Autodesk Inventor part; units mm, degrees
(part 6 of 6)
sketch "スケッチ6" plane through (0, 0, 3) normal (0, 0, 1) x (1, 0, 0)
  arc A0 (23.1244, 53.4347) -> (21.933, 55.8475) centre (21.2019, 53.9859) ccw projected
  arc A1 (21.933, 55.8475) -> (10.9945, 58.9841) centre (0, 0) ccw projected
  arc A2 (10.9945, 58.9841) -> (8.7055, 57.5692) centre (10.628, 57.0179) ccw projected
  line L0 (8.7055, 57.5692) -> (4.5912, 43.221) projected
  arc A3 (3.3812, 41.9035) -> (4.5912, 43.221) centre (2.6687, 43.7723) ccw projected
  line L1 (3.3812, 41.9035) -> (-9.7193, 36.9085) projected
  arc A4 (-12.3349, 38.1621) -> (-9.7193, 36.9085) centre (-10.4318, 38.7772) ccw projected
  line L2 (-12.3349, 38.1621) -> (-15.32, 47.3978) projected
  line L3 (-15.32, 47.3978) -> (-15.6651, 47.2849) projected
  line L4 (-15.6651, 47.2849) -> (-16.0093, 47.1694) projected
  line L5 (-16.0093, 47.1694) -> (-16.3527, 47.0515) projected
  line L6 (-16.3527, 47.0515) -> (-16.6952, 46.9311) projected
  line L7 (-16.6952, 46.9311) -> (-17.0368, 46.8081) projected
  line L8 (-17.0368, 46.8081) -> (-17.3775, 46.6827) projected
  line L9 (-17.3775, 46.6827) -> (-17.7172, 46.5548) projected
  line L10 (-17.7172, 46.5548) -> (-18.0561, 46.4245) projected
  line L11 (-18.0561, 46.4245) -> (-18.394, 46.2916) projected
  line L12 (-18.394, 46.2916) -> (-18.7309, 46.1563) projected
  line L13 (-18.7309, 46.1563) -> (-18.8024, 45.721) projected
  line L14 (-18.8024, 45.721) -> (-18.866, 45.2878) projected
  line L15 (-18.866, 45.2878) -> (-18.9216, 44.8569) projected
  line L16 (-18.9216, 44.8569) -> (-18.969, 44.4283) projected
  line L17 (-18.969, 44.4283) -> (-19.0083, 44.0023) projected
  line L18 (-19.0083, 44.0023) -> (-19.0392, 43.579) projected
  line L19 (-19.0392, 43.579) -> (-19.0617, 43.1585) projected
  line L20 (-19.0617, 43.1585) -> (-19.0757, 42.7409) projected
  line L21 (-19.0757, 42.7409) -> (-19.081, 42.3265) projected
  line L22 (-19.081, 42.3265) -> (-19.0774, 41.9154) projected
  line L23 (-19.0774, 41.9154) -> (-19.0647, 41.5079) projected
  line L24 (-19.0647, 41.5079) -> (-19.0425, 41.1041) projected
  line L25 (-19.0425, 41.1041) -> (-19.0107, 40.7043) projected
  line L26 (-19.0107, 40.7043) -> (-18.9686, 40.3088) projected
  line L27 (-18.9686, 40.3088) -> (-18.9158, 39.9179) projected
  line L28 (-18.9158, 39.9179) -> (-18.8516, 39.5322) projected
  line L29 (-18.8516, 39.5322) -> (-18.7748, 39.1522) projected
  line L30 (-18.7748, 39.1522) -> (-18.6839, 38.7788) projected
  line L31 (-18.6839, 38.7788) -> (-18.576, 38.4134) projected
  line L32 (-18.576, 38.4134) -> (-18.4431, 38.0601) projected
  line L33 (-18.4431, 38.0601) -> (-18.3313, 37.804) projected
  line L34 (-18.3313, 37.804) -> (-18.2337, 37.5507) projected
  line L35 (-18.2337, 37.5507) -> (-18.1486, 37.3012) projected
  line L36 (-18.1486, 37.3012) -> (-18.0734, 37.0569) projected
  line L37 (-18.0734, 37.0569) -> (-18.0133, 36.8155) projected
  line L38 (-18.0133, 36.8155) -> (-17.9685, 36.5772) projected
  line L39 (-17.9685, 36.5772) -> (-17.9393, 36.342) projected
  line L40 (-17.9393, 36.342) -> (-17.9202, 36.1129) projected
  line L41 (-17.9202, 36.1129) -> (-17.9169, 35.8874) projected
  line L42 (-17.9169, 35.8874) -> (-17.9314, 35.6648) projected
  line L43 (-17.9314, 35.6648) -> (-17.9574, 35.4486) projected
  line L44 (-17.9574, 35.4486) -> (-18.0008, 35.2362) projected
  line L45 (-18.0008, 35.2362) -> (-18.0614, 35.0282) projected
  line L46 (-18.0614, 35.0282) -> (-18.1365, 34.8267) projected
  line L47 (-18.1365, 34.8267) -> (-18.2329, 34.6288) projected
  line L48 (-18.2329, 34.6288) -> (-18.3447, 34.4386) projected
  line L49 (-18.3447, 34.4386) -> (-18.4826, 34.2517) projected
  line L50 (-18.4826, 34.2517) -> (-18.6427, 34.0722) projected
  line L51 (-18.6427, 34.0722) -> (-18.8473, 33.8913) projected
  line L52 (-18.8473, 33.8913) -> (-19.1345, 33.6962) projected
  line L53 (-19.1345, 33.6962) -> (-19.1827, 33.6688) projected
  line L54 (-19.1827, 33.6688) -> (-19.2308, 33.6413) projected
  line L55 (-19.2308, 33.6413) -> (-19.2789, 33.6138) projected
  line L56 (-19.2789, 33.6138) -> (-19.327, 33.5862) projected
  line L57 (-19.327, 33.5862) -> (-19.375, 33.5585) projected
  line L58 (-19.375, 33.5585) -> (-19.423, 33.5307) projected
  line L59 (-19.423, 33.5307) -> (-19.4709, 33.5029) projected
  line L60 (-19.4709, 33.5029) -> (-19.5188, 33.475) projected
  line L61 (-19.5188, 33.475) -> (-19.5667, 33.4471) projected
  line L62 (-19.5667, 33.4471) -> (-19.6145, 33.4191) projected
  line L63 (-19.6145, 33.4191) -> (-19.9271, 33.2679) projected
  line L64 (-19.9271, 33.2679) -> (-20.186, 33.1812) projected
  line L65 (-20.186, 33.1812) -> (-20.4215, 33.1323) projected
  line L66 (-20.4215, 33.1323) -> (-20.6524, 33.1063) projected
  line L67 (-20.6524, 33.1063) -> (-20.8729, 33.1046) projected
  line L68 (-20.8729, 33.1046) -> (-21.0926, 33.12) projected
  line L69 (-21.0926, 33.12) -> (-21.3046, 33.1558) projected
  line L70 (-21.3046, 33.1558) -> (-21.515, 33.2073) projected
  line L71 (-21.515, 33.2073) -> (-21.7207, 33.2758) projected
  line L72 (-21.7207, 33.2758) -> (-21.9209, 33.3615) projected
  line L73 (-21.9209, 33.3615) -> (-22.121, 33.4602) projected
  line L74 (-22.121, 33.4602) -> (-22.3146, 33.5758) projected
  line L75 (-22.3146, 33.5758) -> (-22.5034, 33.7069) projected
  line L76 (-22.5034, 33.7069) -> (-22.6925, 33.8498) projected
  line L77 (-22.6925, 33.8498) -> (-22.8765, 34.0078) projected
  line L78 (-22.8765, 34.0078) -> (-23.0555, 34.1805) projected
  line L79 (-23.0555, 34.1805) -> (-23.2294, 34.3678) projected
  line L80 (-23.2294, 34.3678) -> (-23.403, 34.5662) projected
  line L81 (-23.403, 34.5662) -> (-23.5736, 34.7774) projected
  line L82 (-23.5736, 34.7774) -> (-23.7394, 35.0022) projected
  line L83 (-23.7394, 35.0022) -> (-23.979, 35.294) projected
  line L84 (-23.979, 35.294) -> (-24.2415, 35.5701) projected
  line L85 (-24.2415, 35.5701) -> (-24.5194, 35.8356) projected
  line L86 (-24.5194, 35.8356) -> (-24.8101, 36.092) projected
  line L87 (-24.8101, 36.092) -> (-25.1121, 36.3405) projected
  line L88 (-25.1121, 36.3405) -> (-25.4241, 36.5817) projected
  line L89 (-25.4241, 36.5817) -> (-25.7456, 36.8158) projected
  line L90 (-25.7456, 36.8158) -> (-26.0759, 37.0434) projected
  line L91 (-26.0759, 37.0434) -> (-26.4145, 37.2644) projected
  line L92 (-26.4145, 37.2644) -> (-26.7611, 37.4792) projected
  line L93 (-26.7611, 37.4792) -> (-27.1153, 37.6879) projected
  line L94 (-27.1153, 37.6879) -> (-27.4768, 37.8905) projected
  line L95 (-27.4768, 37.8905) -> (-27.8455, 38.0872) projected
  line L96 (-27.8455, 38.0872) -> (-28.2209, 38.2779) projected
  line L97 (-28.2209, 38.2779) -> (-28.603, 38.4628) projected
  line L98 (-28.603, 38.4628) -> (-28.9916, 38.6418) projected
  line L99 (-28.9916, 38.6418) -> (-29.3864, 38.815) projected
  line L100 (-29.3864, 38.815) -> (-29.7874, 38.9823) projected
  line L101 (-29.7874, 38.9823) -> (-30.1943, 39.1439) projected
  line L102 (-30.1943, 39.1439) -> (-30.6071, 39.2996) projected
  line L103 (-30.6071, 39.2996) -> (-30.8927, 39.0755) projected
  line L104 (-30.8927, 39.0755) -> (-31.1767, 38.8493) projected
  line L105 (-31.1767, 38.8493) -> (-31.459, 38.621) projected
  line L106 (-31.459, 38.621) -> (-31.7397, 38.3907) projected
  line L107 (-31.7397, 38.3907) -> (-32.0186, 38.1583) projected
  line L108 (-32.0186, 38.1583) -> (-32.2959, 37.924) projected
  line L109 (-32.2959, 37.924) -> (-32.5715, 37.6876) projected
  line L110 (-32.5715, 37.6876) -> (-32.8453, 37.4492) projected
  line L111 (-32.8453, 37.4492) -> (-33.1173, 37.2088) projected
  line L112 (-33.1173, 37.2088) -> (-33.3877, 36.9664) projected
  line L113 (-33.3877, 36.9664) -> (-33.306, 36.5329) projected
  line L114 (-33.306, 36.5329) -> (-33.2176, 36.1041) projected
  line L115 (-33.2176, 36.1041) -> (-33.1224, 35.6801) projected
  line L116 (-33.1224, 35.6801) -> (-33.0204, 35.2612) projected
  line L117 (-33.0204, 35.2612) -> (-32.9116, 34.8475) projected
  line L118 (-32.9116, 34.8475) -> (-32.7959, 34.4391) projected
  line L119 (-32.7959, 34.4391) -> (-32.6732, 34.0362) projected
  line L120 (-32.6732, 34.0362) -> (-32.5436, 33.639) projected
  line L121 (-32.5436, 33.639) -> (-32.4068, 33.2478) projected
  line L122 (-32.4068, 33.2478) -> (-32.2628, 32.8628) projected
  line L123 (-32.2628, 32.8628) -> (-32.1115, 32.4841) projected
  line L124 (-32.1115, 32.4841) -> (-31.9525, 32.1123) projected
  line L125 (-31.9525, 32.1123) -> (-31.7858, 31.7475) projected
  line L126 (-31.7858, 31.7475) -> (-31.6111, 31.3902) projected
  line L127 (-31.6111, 31.3902) -> (-31.4278, 31.041) projected
  line L128 (-31.4278, 31.041) -> (-31.2355, 30.7005) projected
  line L129 (-31.2355, 30.7005) -> (-31.0334, 30.3697) projected
  line L130 (-31.0334, 30.3697) -> (-30.8202, 30.0499) projected
  line L131 (-30.8202, 30.0499) -> (-30.5939, 29.7434) projected
  line L132 (-30.5939, 29.7434) -> (-30.3482, 29.4569) projected
  line L133 (-30.3482, 29.4569) -> (-30.1555, 29.2545) projected
  line L134 (-30.1555, 29.2545) -> (-29.9772, 29.0498) projected
  line L135 (-29.9772, 29.0498) -> (-29.8119, 28.8444) projected
  line L136 (-29.8119, 28.8444) -> (-29.6577, 28.6406) projected
  line L137 (-29.6577, 28.6406) -> (-29.5186, 28.4343) projected
  line L138 (-29.5186, 28.4343) -> (-29.395, 28.2257) projected
  line L139 (-29.395, 28.2257) -> (-29.2872, 28.0147) projected
  line L140 (-29.2872, 28.0147) -> (-29.1908, 27.806) projected
  line L141 (-29.1908, 27.806) -> (-29.1106, 27.5952) projected
  line L142 (-29.1106, 27.5952) -> (-29.0481, 27.381) projected
  line L143 (-29.0481, 27.381) -> (-28.9985, 27.169) projected
  line L144 (-28.9985, 27.169) -> (-28.9667, 26.9545) projected
  line L145 (-28.9667, 26.9545) -> (-28.9525, 26.7384) projected
  line L146 (-28.9525, 26.7384) -> (-28.9541, 26.5234) projected
  line L147 (-28.9541, 26.5234) -> (-28.9771, 26.3044) projected
  line L148 (-28.9771, 26.3044) -> (-29.0171, 26.0875) projected
  line L149 (-29.0171, 26.0875) -> (-29.0828, 25.8646) projected
  line L150 (-29.0828, 25.8646) -> (-29.1718, 25.6412) projected
  line L151 (-29.1718, 25.6412) -> (-29.3021, 25.4012) projected
  line L152 (-29.3021, 25.4012) -> (-29.5054, 25.1196) projected
  line L153 (-29.5054, 25.1196) -> (-29.5412, 25.0774) projected
  line L154 (-29.5412, 25.0774) -> (-29.5771, 25.0351) projected
  line L155 (-29.5771, 25.0351) -> (-29.6129, 24.9928) projected
  line L156 (-29.6129, 24.9928) -> (-29.6486, 24.9504) projected
  line L157 (-29.6486, 24.9504) -> (-29.6842, 24.908) projected
  line L158 (-29.6842, 24.908) -> (-29.7198, 24.8655) projected
  line L159 (-29.7198, 24.8655) -> (-29.7553, 24.823) projected
  line L160 (-29.7553, 24.823) -> (-29.7908, 24.7804) projected
  line L161 (-29.7908, 24.7804) -> (-29.8262, 24.7378) projected
  line L162 (-29.8262, 24.7378) -> (-29.8616, 24.6951) projected
  line L163 (-29.8616, 24.6951) -> (-30.1036, 24.4461) projected
  line L164 (-30.1036, 24.4461) -> (-30.3173, 24.2761) projected
  line L165 (-30.3173, 24.2761) -> (-30.5219, 24.1496) projected
  line L166 (-30.5219, 24.1496) -> (-30.7299, 24.0462) projected
  line L167 (-30.7299, 24.0462) -> (-30.9366, 23.9692) projected
  line L168 (-30.9366, 23.9692) -> (-31.1483, 23.9085) projected
  line L169 (-31.1483, 23.9085) -> (-31.3597, 23.8696) projected
  line L170 (-31.3597, 23.8696) -> (-31.575, 23.8461) projected
  line L171 (-31.575, 23.8461) -> (-31.7918, 23.8401) projected
  line L172 (-31.7918, 23.8401) -> (-32.0092, 23.8521) projected
  line L173 (-32.0092, 23.8521) -> (-32.231, 23.8765) projected
  line L174 (-32.231, 23.8765) -> (-32.4525, 23.9189) projected
  line L175 (-32.4525, 23.9189) -> (-32.6748, 23.9775) projected
  line L176 (-32.6748, 23.9775) -> (-32.9013, 24.0471) projected
  line L177 (-32.9013, 24.0471) -> (-33.1282, 24.1326) projected
  line L178 (-33.1282, 24.1326) -> (-33.3555, 24.2337) projected
  line L179 (-33.3555, 24.2337) -> (-33.583, 24.3502) projected
  line L180 (-33.583, 24.3502) -> (-33.814, 24.4773) projected
  line L181 (-33.814, 24.4773) -> (-34.0465, 24.6174) projected
  line L182 (-34.0465, 24.6174) -> (-34.2792, 24.772) projected
  line L183 (-34.2792, 24.772) -> (-34.6041, 24.9642) projected
  line L184 (-34.6041, 24.9642) -> (-34.9452, 25.1339) projected
  line L185 (-34.9452, 25.1339) -> (-35.2972, 25.2883) projected
  line L186 (-35.2972, 25.2883) -> (-35.6581, 25.4299) projected
  line L187 (-35.6581, 25.4299) -> (-36.0268, 25.5601) projected
  line L188 (-36.0268, 25.5601) -> (-36.4025, 25.68) projected
  line L189 (-36.4025, 25.68) -> (-36.7847, 25.7901) projected
  line L190 (-36.7847, 25.7901) -> (-37.1729, 25.8909) projected
  line L191 (-37.1729, 25.8909) -> (-37.5667, 25.9828) projected
  line L192 (-37.5667, 25.9828) -> (-37.9659, 26.0661) projected
  line L193 (-37.9659, 26.0661) -> (-38.3701, 26.1411) projected
  line L194 (-38.3701, 26.1411) -> (-38.7791, 26.2078) projected
  line L195 (-38.7791, 26.2078) -> (-39.1928, 26.2665) projected
  line L196 (-39.1928, 26.2665) -> (-39.6108, 26.3174) projected
  line L197 (-39.6108, 26.3174) -> (-40.0331, 26.3604) projected
  line L198 (-40.0331, 26.3604) -> (-40.4594, 26.3957) projected
  line L199 (-40.4594, 26.3957) -> (-40.8897, 26.4234) projected
  line L200 (-40.8897, 26.4234) -> (-41.3237, 26.4435) projected
  line L201 (-41.3237, 26.4435) -> (-41.7614, 26.4561) projected
  line L202 (-41.7614, 26.4561) -> (-42.2025, 26.4613) projected
  line L203 (-42.2025, 26.4613) -> (-42.3943, 26.153) projected
  line L204 (-42.3943, 26.153) -> (-42.5838, 25.8433) projected
  line L205 (-42.5838, 25.8433) -> (-42.771, 25.5322) projected
  line L206 (-42.771, 25.5322) -> (-42.9559, 25.2198) projected
  line L207 (-42.9559, 25.2198) -> (-43.1386, 24.9061) projected
  line L208 (-43.1386, 24.9061) -> (-43.319, 24.591) projected
  line L209 (-43.319, 24.591) -> (-43.4971, 24.2746) projected
  line L210 (-43.4971, 24.2746) -> (-43.6728, 23.957) projected
  line L211 (-43.6728, 23.957) -> (-43.8463, 23.638) projected
  line L212 (-43.8463, 23.638) -> (-44.0174, 23.3178) projected
  line L213 (-44.0174, 23.3178) -> (-43.7924, 22.9383) projected
  line L214 (-43.7924, 22.9383) -> (-43.5626, 22.5656) projected
  line L215 (-43.5626, 22.5656) -> (-43.3282, 22.1998) projected
  line L216 (-43.3282, 22.1998) -> (-43.0891, 21.841) projected
  line L217 (-43.0891, 21.841) -> (-42.8453, 21.4895) projected
  line L218 (-42.8453, 21.4895) -> (-42.5969, 21.1453) projected
  line L219 (-42.5969, 21.1453) -> (-42.3439, 20.8086) projected
  line L220 (-42.3439, 20.8086) -> (-42.0862, 20.4798) projected
  line L221 (-42.0862, 20.4798) -> (-41.8239, 20.1589) projected
  line L222 (-41.8239, 20.1589) -> (-41.5569, 19.8464) projected
  line L223 (-41.5569, 19.8464) -> (-41.2851, 19.5423) projected
  line L224 (-41.2851, 19.5423) -> (-41.0086, 19.2472) projected
  line L225 (-41.0086, 19.2472) -> (-40.7272, 18.9615) projected
  line L226 (-40.7272, 18.9615) -> (-40.4408, 18.6855) projected
  line L227 (-40.4408, 18.6855) -> (-40.1491, 18.4201) projected
  line L228 (-40.1491, 18.4201) -> (-39.852, 18.1659) projected
  line L229 (-39.852, 18.1659) -> (-39.5489, 17.9241) projected
  line L230 (-39.5489, 17.9241) -> (-39.2392, 17.6965) projected
  line L231 (-39.2392, 17.6965) -> (-38.9217, 17.4859) projected
  line L232 (-38.9217, 17.4859) -> (-38.5928, 17.3007) projected
  line L233 (-38.5928, 17.3007) -> (-38.3425, 17.1764) projected
  line L234 (-38.3425, 17.1764) -> (-38.105, 17.0451) projected
  line L235 (-38.105, 17.0451) -> (-37.8794, 16.9086) projected
  line L236 (-37.8794, 16.9086) -> (-37.6648, 16.7698) projected
  line L237 (-37.6648, 16.7698) -> (-37.4636, 16.6236) projected
  line L238 (-37.4636, 16.6236) -> (-37.2761, 16.4698) projected
  line L239 (-37.2761, 16.4698) -> (-37.1025, 16.3084) projected
  line L240 (-37.1025, 16.3084) -> (-36.9406, 16.1452) projected
  line L241 (-36.9406, 16.1452) -> (-36.7931, 15.9746) projected
  line L242 (-36.7931, 15.9746) -> (-36.6611, 15.7947) projected
  line L243 (-36.6611, 15.7947) -> (-36.5421, 15.6124) projected
  line L244 (-36.5421, 15.6124) -> (-36.4388, 15.4218) projected
  line L245 (-36.4388, 15.4218) -> (-36.3516, 15.2235) projected
  line L246 (-36.3516, 15.2235) -> (-36.2795, 15.0209) projected
  line L247 (-36.2795, 15.0209) -> (-36.2262, 14.8073) projected
  line L248 (-36.2262, 14.8073) -> (-36.1896, 14.5898) projected
  line L249 (-36.1896, 14.5898) -> (-36.1751, 14.3579) projected
  line L250 (-36.1751, 14.3579) -> (-36.1824, 14.1175) projected
  line L251 (-36.1824, 14.1175) -> (-36.2227, 13.8474) projected
  line L252 (-36.2227, 13.8474) -> (-36.3174, 13.5133) projected
  line L253 (-36.3174, 13.5133) -> (-36.3367, 13.4614) projected
  line L254 (-36.3367, 13.4614) -> (-36.3559, 13.4094) projected
  line L255 (-36.3559, 13.4094) -> (-36.375, 13.3574) projected
  line L256 (-36.375, 13.3574) -> (-36.3941, 13.3053) projected
  line L257 (-36.3941, 13.3053) -> (-36.4131, 13.2533) projected
  line L258 (-36.4131, 13.2533) -> (-36.432, 13.2012) projected
  line L259 (-36.432, 13.2012) -> (-36.4508, 13.1491) projected
  line L260 (-36.4508, 13.1491) -> (-36.4696, 13.0969) projected
  line L261 (-36.4696, 13.0969) -> (-36.4883, 13.0448) projected
  line L262 (-36.4883, 13.0448) -> (-36.5069, 12.9926) projected
  line L263 (-36.5069, 12.9926) -> (-36.6492, 12.6758) projected
  line L264 (-36.6492, 12.6758) -> (-36.7919, 12.4429) projected
  line L265 (-36.7919, 12.4429) -> (-36.9408, 12.2541) projected
  line L266 (-36.9408, 12.2541) -> (-37.1009, 12.0858) projected
  line L267 (-37.1009, 12.0858) -> (-37.2688, 11.9427) projected
  line L268 (-37.2688, 11.9427) -> (-37.447, 11.8133) projected
  line L269 (-37.447, 11.8133) -> (-37.6324, 11.7044) projected
  line L270 (-37.6324, 11.7044) -> (-37.8267, 11.6087) projected
  line L271 (-37.8267, 11.6087) -> (-38.0283, 11.529) projected
  line L272 (-38.0283, 11.529) -> (-38.2367, 11.4659) projected
  line L273 (-38.2367, 11.4659) -> (-38.4534, 11.4129) projected
  line L274 (-38.4534, 11.4129) -> (-38.6761, 11.377) projected
  line L275 (-38.6761, 11.377) -> (-38.905, 11.3561) projected
  line L276 (-38.905, 11.3561) -> (-39.1417, 11.344) projected
  line L277 (-39.1417, 11.344) -> (-39.3842, 11.3467) projected
  line L278 (-39.3842, 11.3467) -> (-39.6323, 11.364) projected
  line L279 (-39.6323, 11.364) -> (-39.886, 11.3956) projected
  line L280 (-39.886, 11.3956) -> (-40.1465, 11.4361) projected
  line L281 (-40.1465, 11.4361) -> (-40.4129, 11.4882) projected
  line L282 (-40.4129, 11.4882) -> (-40.6845, 11.5538) projected
  line L283 (-40.6845, 11.5538) -> (-41.0555, 11.6234) projected
  line L284 (-41.0555, 11.6234) -> (-41.4341, 11.6662) projected
  line L285 (-41.4341, 11.6662) -> (-41.8176, 11.6908) projected
  line L286 (-41.8176, 11.6908) -> (-42.2052, 11.7005) projected
  line L287 (-42.2052, 11.7005) -> (-42.5962, 11.6968) projected
  line L288 (-42.5962, 11.6968) -> (-42.9903, 11.6809) projected
  line L289 (-42.9903, 11.6809) -> (-43.387, 11.6536) projected
  line L290 (-43.387, 11.6536) -> (-43.7863, 11.6156) projected
  line L291 (-43.7863, 11.6156) -> (-44.1878, 11.5673) projected
  line L292 (-44.1878, 11.5673) -> (-44.5914, 11.509) projected
  line L293 (-44.5914, 11.509) -> (-44.9969, 11.4412) projected
  line L294 (-44.9969, 11.4412) -> (-45.4041, 11.3641) projected
  line L295 (-45.4041, 11.3641) -> (-45.8128, 11.2778) projected
  line L296 (-45.8128, 11.2778) -> (-46.223, 11.1825) projected
  line L297 (-46.223, 11.1825) -> (-46.6346, 11.0786) projected
  line L298 (-46.6346, 11.0786) -> (-47.0473, 10.9659) projected
  line L299 (-47.0473, 10.9659) -> (-47.4611, 10.8448) projected
  line L300 (-47.4611, 10.8448) -> (-47.8758, 10.7152) projected
  line L301 (-47.8758, 10.7152) -> (-48.2914, 10.5774) projected
  line L302 (-48.2914, 10.5774) -> (-48.7077, 10.4313) projected
  line L303 (-48.7077, 10.4313) -> (-48.7824, 10.0761) projected
  line L304 (-48.7824, 10.0761) -> (-48.8546, 9.7203) projected
  line L305 (-48.8546, 9.7203) -> (-48.9241, 9.3639) projected
  line L306 (-48.9241, 9.3639) -> (-48.9911, 9.0071) projected
  line L307 (-48.9911, 9.0071) -> (-49.0554, 8.6498) projected
  line L308 (-49.0554, 8.6498) -> (-49.1172, 8.292) projected
  line L309 (-49.1172, 8.292) -> (-49.1763, 7.9338) projected
  line L310 (-49.1763, 7.9338) -> (-49.2328, 7.5752) projected
  line L311 (-49.2328, 7.5752) -> (-49.2867, 7.2162) projected
  line L312 (-49.2867, 7.2162) -> (-49.338, 6.8568) projected
  line L313 (-49.338, 6.8568) -> (-48.9968, 6.5771) projected
  line L314 (-48.9968, 6.5771) -> (-48.6534, 6.3055) projected
  line L315 (-48.6534, 6.3055) -> (-48.308, 6.0419) projected
  line L316 (-48.308, 6.0419) -> (-47.9606, 5.7865) projected
  line L317 (-47.9606, 5.7865) -> (-47.6113, 5.5395) projected
  line L318 (-47.6113, 5.5395) -> (-47.2601, 5.3011) projected
  line L319 (-47.2601, 5.3011) -> (-46.9072, 5.0713) projected
  line L320 (-46.9072, 5.0713) -> (-46.5526, 4.8504) projected
  line L321 (-46.5526, 4.8504) -> (-46.1963, 4.6386) projected
  line L322 (-46.1963, 4.6386) -> (-45.8385, 4.4362) projected
  line L323 (-45.8385, 4.4362) -> (-45.4792, 4.2434) projected
  line L324 (-45.4792, 4.2434) -> (-45.1184, 4.0607) projected
  line L325 (-45.1184, 4.0607) -> (-44.7563, 3.8884) projected
  line L326 (-44.7563, 3.8884) -> (-44.3927, 3.7271) projected
  line L327 (-44.3927, 3.7271) -> (-44.0279, 3.5774) projected
  line L328 (-44.0279, 3.5774) -> (-43.6617, 3.4402) projected
  line L329 (-43.6617, 3.4402) -> (-43.2942, 3.3167) projected
  line L330 (-43.2942, 3.3167) -> (-42.9254, 3.2087) projected
  line L331 (-42.9254, 3.2087) -> (-42.555, 3.1194) projected
  line L332 (-42.555, 3.1194) -> (-42.1825, 3.0578) projected
  line L333 (-42.1825, 3.0578) -> (-41.9049, 3.0266) projected
  line L334 (-41.9049, 3.0266) -> (-41.6367, 2.9845) projected
  line L335 (-41.6367, 2.9845) -> (-41.3781, 2.9334) projected
  line L336 (-41.3781, 2.9334) -> (-41.1289, 2.8764) projected
  line L337 (-41.1289, 2.8764) -> (-40.8898, 2.8078) projected
  line L338 (-40.8898, 2.8078) -> (-40.661, 2.7274) projected
  line L339 (-40.661, 2.7274) -> (-40.4428, 2.6351) projected
  line L340 (-40.4428, 2.6351) -> (-40.2348, 2.5371) projected
  line L341 (-40.2348, 2.5371) -> (-40.0379, 2.4272) projected
  line L342 (-40.0379, 2.4272) -> (-39.8523, 2.3033) projected
  line L343 (-39.8523, 2.3033) -> (-39.6781, 2.1727) projected
  line L344 (-39.6781, 2.1727) -> (-39.5158, 2.0289) projected
  line L345 (-39.5158, 2.0289) -> (-39.366, 1.8725) projected
  line L346 (-39.366, 1.8725) -> (-39.2291, 1.7067) projected
  line L347 (-39.2291, 1.7067) -> (-39.1059, 1.5242) projected
  line L348 (-39.1059, 1.5242) -> (-38.997, 1.3323) projected
  line L349 (-38.997, 1.3323) -> (-38.9042, 1.1194) projected
  line L350 (-38.9042, 1.1194) -> (-38.8288, 0.891) projected
  line L351 (-38.8288, 0.891) -> (-38.7743, 0.6234) projected
  line L352 (-38.7743, 0.6234) -> (-38.749, 0.2771) projected
  line L353 (-38.749, 0.2771) -> (-38.7494, 0.2217) projected
  line L354 (-38.7494, 0.2217) -> (-38.7496, 0.1663) projected
  line L355 (-38.7496, 0.1663) -> (-38.7498, 0.1108) projected
  line L356 (-38.7498, 0.1108) -> (-38.75, 0.0554) projected
  line L357 (-38.75, 0.0554) -> (-38.75, 0) projected
  line L358 (-38.75, 0) -> (-38.75, -0.0554) projected
  line L359 (-38.75, -0.0554) -> (-38.7498, -0.1108) projected
  line L360 (-38.7498, -0.1108) -> (-38.7496, -0.1663) projected
  line L361 (-38.7496, -0.1663) -> (-38.7494, -0.2217) projected
  line L362 (-38.7494, -0.2217) -> (-38.749, -0.2771) projected
  line L363 (-38.749, -0.2771) -> (-38.7743, -0.6234) projected
  line L364 (-38.7743, -0.6234) -> (-38.8288, -0.891) projected
  line L365 (-38.8288, -0.891) -> (-38.9042, -1.1194) projected
  line L366 (-38.9042, -1.1194) -> (-38.997, -1.3323) projected
  line L367 (-38.997, -1.3323) -> (-39.1059, -1.5242) projected
  line L368 (-39.1059, -1.5242) -> (-39.2291, -1.7067) projected
  line L369 (-39.2291, -1.7067) -> (-39.366, -1.8725) projected
  line L370 (-39.366, -1.8725) -> (-39.5158, -2.0289) projected
  line L371 (-39.5158, -2.0289) -> (-39.6781, -2.1727) projected
  line L372 (-39.6781, -2.1727) -> (-39.8523, -2.3033) projected
  line L373 (-39.8523, -2.3033) -> (-40.0379, -2.4272) projected
  line L374 (-40.0379, -2.4272) -> (-40.2348, -2.5371) projected
  line L375 (-40.2348, -2.5371) -> (-40.4428, -2.6351) projected
  line L376 (-40.4428, -2.6351) -> (-40.661, -2.7274) projected
  line L377 (-40.661, -2.7274) -> (-40.8898, -2.8078) projected
  line L378 (-40.8898, -2.8078) -> (-41.1289, -2.8764) projected
  line L379 (-41.1289, -2.8764) -> (-41.3781, -2.9334) projected
  line L380 (-41.3781, -2.9334) -> (-41.6367, -2.9845) projected
  line L381 (-41.6367, -2.9845) -> (-41.9049, -3.0266) projected
  line L382 (-41.9049, -3.0266) -> (-42.1825, -3.0578) projected
  line L383 (-42.1825, -3.0578) -> (-42.555, -3.1194) projected
  line L384 (-42.555, -3.1194) -> (-42.9254, -3.2087) projected
  line L385 (-42.9254, -3.2087) -> (-43.2942, -3.3167) projected
  line L386 (-43.2942, -3.3167) -> (-43.6617, -3.4402) projected
  line L387 (-43.6617, -3.4402) -> (-44.0279, -3.5774) projected
  line L388 (-44.0279, -3.5774) -> (-44.3927, -3.7271) projected
  line L389 (-44.3927, -3.7271) -> (-44.7563, -3.8884) projected
  line L390 (-44.7563, -3.8884) -> (-45.1184, -4.0607) projected
  line L391 (-45.1184, -4.0607) -> (-45.4792, -4.2434) projected
  line L392 (-45.4792, -4.2434) -> (-45.8385, -4.4362) projected
  line L393 (-45.8385, -4.4362) -> (-46.1963, -4.6386) projected
  line L394 (-46.1963, -4.6386) -> (-46.5526, -4.8504) projected
  line L395 (-46.5526, -4.8504) -> (-46.9072, -5.0713) projected
  line L396 (-46.9072, -5.0713) -> (-47.2601, -5.3011) projected
  line L397 (-47.2601, -5.3011) -> (-47.6113, -5.5395) projected
  line L398 (-47.6113, -5.5395) -> (-47.9606, -5.7865) projected
  line L399 (-47.9606, -5.7865) -> (-48.308, -6.0419) projected
  line L400 (-48.308, -6.0419) -> (-48.6534, -6.3055) projected
  line L401 (-48.6534, -6.3055) -> (-48.9968, -6.5771) projected
  line L402 (-48.9968, -6.5771) -> (-49.338, -6.8568) projected
  line L403 (-49.338, -6.8568) -> (-49.2867, -7.2162) projected
  line L404 (-49.2867, -7.2162) -> (-49.2328, -7.5752) projected
  line L405 (-49.2328, -7.5752) -> (-49.1763, -7.9338) projected
  line L406 (-49.1763, -7.9338) -> (-49.1172, -8.292) projected
  line L407 (-49.1172, -8.292) -> (-49.0554, -8.6498) projected
  line L408 (-49.0554, -8.6498) -> (-48.9911, -9.0071) projected
  line L409 (-48.9911, -9.0071) -> (-48.9241, -9.3639) projected
  line L410 (-48.9241, -9.3639) -> (-48.8546, -9.7203) projected
  line L411 (-48.8546, -9.7203) -> (-48.7824, -10.0761) projected
  line L412 (-48.7824, -10.0761) -> (-48.7077, -10.4313) projected
  line L413 (-48.7077, -10.4313) -> (-48.2914, -10.5774) projected
  line L414 (-48.2914, -10.5774) -> (-47.8758, -10.7152) projected
  line L415 (-47.8758, -10.7152) -> (-47.4611, -10.8448) projected
  line L416 (-47.4611, -10.8448) -> (-47.0473, -10.9659) projected
  line L417 (-47.0473, -10.9659) -> (-46.6346, -11.0786) projected
  line L418 (-46.6346, -11.0786) -> (-46.223, -11.1825) projected
  line L419 (-46.223, -11.1825) -> (-45.8128, -11.2778) projected
  line L420 (-45.8128, -11.2778) -> (-45.4041, -11.3641) projected
  line L421 (-45.4041, -11.3641) -> (-44.9969, -11.4412) projected
  line L422 (-44.9969, -11.4412) -> (-44.5914, -11.509) projected
  line L423 (-44.5914, -11.509) -> (-44.1878, -11.5673) projected
  line L424 (-44.1878, -11.5673) -> (-43.7863, -11.6156) projected
  line L425 (-43.7863, -11.6156) -> (-43.387, -11.6536) projected
  line L426 (-43.387, -11.6536) -> (-42.9903, -11.6809) projected
  line L427 (-42.9903, -11.6809) -> (-42.5962, -11.6968) projected
  line L428 (-42.5962, -11.6968) -> (-42.2052, -11.7005) projected
  line L429 (-42.2052, -11.7005) -> (-41.8176, -11.6908) projected
  line L430 (-41.8176, -11.6908) -> (-41.4341, -11.6662) projected
  line L431 (-41.4341, -11.6662) -> (-41.0555, -11.6234) projected
  line L432 (-41.0555, -11.6234) -> (-40.6845, -11.5538) projected
  line L433 (-40.6845, -11.5538) -> (-40.4129, -11.4882) projected
  line L434 (-40.4129, -11.4882) -> (-40.1465, -11.4361) projected
  line L435 (-40.1465, -11.4361) -> (-39.886, -11.3956) projected
  line L436 (-39.886, -11.3956) -> (-39.6323, -11.364) projected
  line L437 (-39.6323, -11.364) -> (-39.3842, -11.3467) projected
  line L438 (-39.3842, -11.3467) -> (-39.1417, -11.344) projected
  line L439 (-39.1417, -11.344) -> (-38.905, -11.3561) projected
  line L440 (-38.905, -11.3561) -> (-38.6761, -11.377) projected
  line L441 (-38.6761, -11.377) -> (-38.4534, -11.4129) projected
  line L442 (-38.4534, -11.4129) -> (-38.2367, -11.4659) projected
  line L443 (-38.2367, -11.4659) -> (-38.0283, -11.529) projected
  line L444 (-38.0283, -11.529) -> (-37.8267, -11.6087) projected
  line L445 (-37.8267, -11.6087) -> (-37.6324, -11.7044) projected
  line L446 (-37.6324, -11.7044) -> (-37.447, -11.8133) projected
  line L447 (-37.447, -11.8133) -> (-37.2688, -11.9427) projected
  line L448 (-37.2688, -11.9427) -> (-37.1009, -12.0858) projected
  line L449 (-37.1009, -12.0858) -> (-36.9408, -12.2541) projected
  line L450 (-36.9408, -12.2541) -> (-36.7919, -12.4429) projected
  line L451 (-36.7919, -12.4429) -> (-36.6492, -12.6758) projected
  line L452 (-36.6492, -12.6758) -> (-36.5069, -12.9926) projected
  line L453 (-36.5069, -12.9926) -> (-36.4883, -13.0448) projected
  line L454 (-36.4883, -13.0448) -> (-36.4696, -13.0969) projected
  line L455 (-36.4696, -13.0969) -> (-36.4508, -13.1491) projected
  line L456 (-36.4508, -13.1491) -> (-36.432, -13.2012) projected
  line L457 (-36.432, -13.2012) -> (-36.4131, -13.2533) projected
  line L458 (-36.4131, -13.2533) -> (-36.3941, -13.3053) projected
  line L459 (-36.3941, -13.3053) -> (-36.375, -13.3574) projected
  line L460 (-36.375, -13.3574) -> (-36.3559, -13.4094) projected
  line L461 (-36.3559, -13.4094) -> (-36.3367, -13.4614) projected
  line L462 (-36.3367, -13.4614) -> (-36.3174, -13.5133) projected
  line L463 (-36.3174, -13.5133) -> (-36.2227, -13.8474) projected
  line L464 (-36.2227, -13.8474) -> (-36.1824, -14.1175) projected
  line L465 (-36.1824, -14.1175) -> (-36.1751, -14.3579) projected
  line L466 (-36.1751, -14.3579) -> (-36.1896, -14.5898) projected
  line L467 (-36.1896, -14.5898) -> (-36.2262, -14.8073) projected
  line L468 (-36.2262, -14.8073) -> (-36.2795, -15.0209) projected
  line L469 (-36.2795, -15.0209) -> (-36.3516, -15.2235) projected
  line L470 (-36.3516, -15.2235) -> (-36.4388, -15.4218) projected
  line L471 (-36.4388, -15.4218) -> (-36.5421, -15.6124) projected
  line L472 (-36.5421, -15.6124) -> (-36.6611, -15.7947) projected
  line L473 (-36.6611, -15.7947) -> (-36.7931, -15.9746) projected
  line L474 (-36.7931, -15.9746) -> (-36.9406, -16.1452) projected
  line L475 (-36.9406, -16.1452) -> (-37.1025, -16.3084) projected
  line L476 (-37.1025, -16.3084) -> (-37.2761, -16.4698) projected
  line L477 (-37.2761, -16.4698) -> (-37.4636, -16.6236) projected
  line L478 (-37.4636, -16.6236) -> (-37.6648, -16.7698) projected
  line L479 (-37.6648, -16.7698) -> (-37.8794, -16.9086) projected
  line L480 (-37.8794, -16.9086) -> (-38.105, -17.0451) projected
  line L481 (-38.105, -17.0451) -> (-38.3425, -17.1764) projected
  line L482 (-38.3425, -17.1764) -> (-38.5928, -17.3007) projected
  line L483 (-38.5928, -17.3007) -> (-38.9217, -17.4859) projected
  line L484 (-38.9217, -17.4859) -> (-39.2392, -17.6965) projected
  line L485 (-39.2392, -17.6965) -> (-39.5489, -17.9241) projected
  line L486 (-39.5489, -17.9241) -> (-39.852, -18.1659) projected
  line L487 (-39.852, -18.1659) -> (-40.1491, -18.4201) projected
  line L488 (-40.1491, -18.4201) -> (-40.4408, -18.6855) projected
  line L489 (-40.4408, -18.6855) -> (-40.7272, -18.9615) projected
  line L490 (-40.7272, -18.9615) -> (-41.0086, -19.2472) projected
  line L491 (-41.0086, -19.2472) -> (-41.2851, -19.5423) projected
  line L492 (-41.2851, -19.5423) -> (-41.5569, -19.8464) projected
  line L493 (-41.5569, -19.8464) -> (-41.8239, -20.1589) projected
  line L494 (-41.8239, -20.1589) -> (-42.0862, -20.4798) projected
  line L495 (-42.0862, -20.4798) -> (-42.3439, -20.8086) projected
  line L496 (-42.3439, -20.8086) -> (-42.5969, -21.1453) projected
  line L497 (-42.5969, -21.1453) -> (-42.8453, -21.4895) projected
  line L498 (-42.8453, -21.4895) -> (-43.0891, -21.841) projected
  line L499 (-43.0891, -21.841) -> (-43.3282, -22.1998) projected
  line L500 (-43.3282, -22.1998) -> (-43.5626, -22.5656) projected
  line L501 (-43.5626, -22.5656) -> (-43.7924, -22.9383) projected
  line L502 (-43.7924, -22.9383) -> (-44.0174, -23.3178) projected
  line L503 (-44.0174, -23.3178) -> (-43.8463, -23.638) projected
  line L504 (-43.8463, -23.638) -> (-43.6728, -23.957) projected
  line L505 (-43.6728, -23.957) -> (-43.4971, -24.2746) projected
  line L506 (-43.4971, -24.2746) -> (-43.319, -24.591) projected
  line L507 (-43.319, -24.591) -> (-43.1386, -24.9061) projected
  line L508 (-43.1386, -24.9061) -> (-42.9559, -25.2198) projected
  line L509 (-42.9559, -25.2198) -> (-42.771, -25.5322) projected
  line L510 (-42.771, -25.5322) -> (-42.5838, -25.8433) projected
  line L511 (-42.5838, -25.8433) -> (-42.3943, -26.153) projected
  line L512 (-42.3943, -26.153) -> (-42.2025, -26.4613) projected
  line L513 (-42.2025, -26.4613) -> (-41.7614, -26.4561) projected
  line L514 (-41.7614, -26.4561) -> (-41.3237, -26.4435) projected
  line L515 (-41.3237, -26.4435) -> (-40.8897, -26.4234) projected
  line L516 (-40.8897, -26.4234) -> (-40.4594, -26.3957) projected
  line L517 (-40.4594, -26.3957) -> (-40.0331, -26.3604) projected
  line L518 (-40.0331, -26.3604) -> (-39.6108, -26.3174) projected
  line L519 (-39.6108, -26.3174) -> (-39.1928, -26.2665) projected
  line L520 (-39.1928, -26.2665) -> (-38.7791, -26.2078) projected
  line L521 (-38.7791, -26.2078) -> (-38.3701, -26.1411) projected
  line L522 (-38.3701, -26.1411) -> (-37.9659, -26.0661) projected
  line L523 (-37.9659, -26.0661) -> (-37.5667, -25.9828) projected
  line L524 (-37.5667, -25.9828) -> (-37.1729, -25.8909) projected
  line L525 (-37.1729, -25.8909) -> (-36.7847, -25.7901) projected
  line L526 (-36.7847, -25.7901) -> (-36.4025, -25.68) projected
  line L527 (-36.4025, -25.68) -> (-36.0268, -25.5601) projected
  line L528 (-36.0268, -25.5601) -> (-35.6581, -25.4299) projected
  line L529 (-35.6581, -25.4299) -> (-35.2972, -25.2883) projected
  line L530 (-35.2972, -25.2883) -> (-34.9452, -25.1339) projected
  line L531 (-34.9452, -25.1339) -> (-34.6041, -24.9642) projected
  line L532 (-34.6041, -24.9642) -> (-34.2792, -24.772) projected
  line L533 (-34.2792, -24.772) -> (-34.0465, -24.6174) projected
  line L534 (-34.0465, -24.6174) -> (-33.814, -24.4773) projected
  line L535 (-33.814, -24.4773) -> (-33.583, -24.3502) projected
  line L536 (-33.583, -24.3502) -> (-33.3555, -24.2337) projected
  line L537 (-33.3555, -24.2337) -> (-33.1282, -24.1326) projected
  line L538 (-33.1282, -24.1326) -> (-32.9013, -24.0471) projected
  line L539 (-32.9013, -24.0471) -> (-32.6748, -23.9775) projected
  line L540 (-32.6748, -23.9775) -> (-32.4525, -23.9189) projected
  line L541 (-32.4525, -23.9189) -> (-32.231, -23.8765) projected
  line L542 (-32.231, -23.8765) -> (-32.0092, -23.8521) projected
  line L543 (-32.0092, -23.8521) -> (-31.7918, -23.8401) projected
  line L544 (-31.7918, -23.8401) -> (-31.575, -23.8461) projected
  line L545 (-31.575, -23.8461) -> (-31.3597, -23.8696) projected
  line L546 (-31.3597, -23.8696) -> (-31.1483, -23.9085) projected
  line L547 (-31.1483, -23.9085) -> (-30.9366, -23.9692) projected
  line L548 (-30.9366, -23.9692) -> (-30.7299, -24.0462) projected
  line L549 (-30.7299, -24.0462) -> (-30.5219, -24.1496) projected
  line L550 (-30.5219, -24.1496) -> (-30.3173, -24.2761) projected
  line L551 (-30.3173, -24.2761) -> (-30.1036, -24.4461) projected
  line L552 (-30.1036, -24.4461) -> (-29.8616, -24.6951) projected
  line L553 (-29.8616, -24.6951) -> (-29.8262, -24.7378) projected
  line L554 (-29.8262, -24.7378) -> (-29.7908, -24.7804) projected
  line L555 (-29.7908, -24.7804) -> (-29.7553, -24.823) projected
  line L556 (-29.7553, -24.823) -> (-29.7198, -24.8655) projected
  line L557 (-29.7198, -24.8655) -> (-29.6842, -24.908) projected
  line L558 (-29.6842, -24.908) -> (-29.6486, -24.9504) projected
  line L559 (-29.6486, -24.9504) -> (-29.6129, -24.9928) projected
  line L560 (-29.6129, -24.9928) -> (-29.5771, -25.0351) projected
  line L561 (-29.5771, -25.0351) -> (-29.5412, -25.0774) projected
  line L562 (-29.5412, -25.0774) -> (-29.5054, -25.1196) projected
  line L563 (-29.5054, -25.1196) -> (-29.3021, -25.4012) projected
  line L564 (-29.3021, -25.4012) -> (-29.1718, -25.6412) projected
  line L565 (-29.1718, -25.6412) -> (-29.0828, -25.8646) projected
  line L566 (-29.0828, -25.8646) -> (-29.0171, -26.0875) projected
  line L567 (-29.0171, -26.0875) -> (-28.9771, -26.3044) projected
  line L568 (-28.9771, -26.3044) -> (-28.9541, -26.5234) projected
  line L569 (-28.9541, -26.5234) -> (-28.9525, -26.7384) projected
  line L570 (-28.9525, -26.7384) -> (-28.9667, -26.9545) projected
  line L571 (-28.9667, -26.9545) -> (-28.9985, -27.169) projected
  line L572 (-28.9985, -27.169) -> (-29.0481, -27.381) projected
  line L573 (-29.0481, -27.381) -> (-29.1106, -27.5952) projected
  line L574 (-29.1106, -27.5952) -> (-29.1908, -27.806) projected
  line L575 (-29.1908, -27.806) -> (-29.2872, -28.0147) projected
  line L576 (-29.2872, -28.0147) -> (-29.395, -28.2257) projected
  line L577 (-29.395, -28.2257) -> (-29.5186, -28.4343) projected
  line L578 (-29.5186, -28.4343) -> (-29.6577, -28.6406) projected
  line L579 (-29.6577, -28.6406) -> (-29.8119, -28.8444) projected
  line L580 (-29.8119, -28.8444) -> (-29.9772, -29.0498) projected
  line L581 (-29.9772, -29.0498) -> (-30.1555, -29.2545) projected
  line L582 (-30.1555, -29.2545) -> (-30.3482, -29.4569) projected
  line L583 (-30.3482, -29.4569) -> (-30.5939, -29.7434) projected
  line L584 (-30.5939, -29.7434) -> (-30.8202, -30.0499) projected
  line L585 (-30.8202, -30.0499) -> (-31.0334, -30.3697) projected
  line L586 (-31.0334, -30.3697) -> (-31.2355, -30.7005) projected
  line L587 (-31.2355, -30.7005) -> (-31.4278, -31.041) projected
  line L588 (-31.4278, -31.041) -> (-31.6111, -31.3902) projected
  line L589 (-31.6111, -31.3902) -> (-31.7858, -31.7475) projected
  line L590 (-31.7858, -31.7475) -> (-31.9525, -32.1123) projected
  line L591 (-31.9525, -32.1123) -> (-32.1115, -32.4841) projected
  line L592 (-32.1115, -32.4841) -> (-32.2628, -32.8628) projected
  line L593 (-32.2628, -32.8628) -> (-32.4068, -33.2478) projected
  line L594 (-32.4068, -33.2478) -> (-32.5436, -33.639) projected
  line L595 (-32.5436, -33.639) -> (-32.6732, -34.0362) projected
  line L596 (-32.6732, -34.0362) -> (-32.7959, -34.4391) projected
  line L597 (-32.7959, -34.4391) -> (-32.9116, -34.8475) projected
  line L598 (-32.9116, -34.8475) -> (-33.0204, -35.2612) projected
  line L599 (-33.0204, -35.2612) -> (-33.1224, -35.6801) projected
  line L600 (-33.1224, -35.6801) -> (-33.2176, -36.1041) projected
  line L601 (-33.2176, -36.1041) -> (-33.306, -36.5329) projected
  line L602 (-33.306, -36.5329) -> (-33.3877, -36.9664) projected
  line L603 (-33.3877, -36.9664) -> (-33.1173, -37.2088) projected
  line L604 (-33.1173, -37.2088) -> (-32.8453, -37.4492) projected
  line L605 (-32.8453, -37.4492) -> (-32.5715, -37.6876) projected
  line L606 (-32.5715, -37.6876) -> (-32.2959, -37.924) projected
  line L607 (-32.2959, -37.924) -> (-32.0186, -38.1583) projected
  line L608 (-32.0186, -38.1583) -> (-31.7397, -38.3907) projected
  line L609 (-31.7397, -38.3907) -> (-31.459, -38.621) projected
  line L610 (-31.459, -38.621) -> (-31.1767, -38.8493) projected
  line L611 (-31.1767, -38.8493) -> (-30.8927, -39.0755) projected
  line L612 (-30.8927, -39.0755) -> (-30.6071, -39.2996) projected
  line L613 (-30.6071, -39.2996) -> (-30.1943, -39.1439) projected
  line L614 (-30.1943, -39.1439) -> (-29.7874, -38.9823) projected
  line L615 (-29.7874, -38.9823) -> (-29.3864, -38.815) projected
  line L616 (-29.3864, -38.815) -> (-28.9916, -38.6418) projected
  line L617 (-28.9916, -38.6418) -> (-28.603, -38.4628) projected
  line L618 (-28.603, -38.4628) -> (-28.2209, -38.2779) projected
  line L619 (-28.2209, -38.2779) -> (-27.8455, -38.0872) projected
  line L620 (-27.8455, -38.0872) -> (-27.4768, -37.8905) projected
  line L621 (-27.4768, -37.8905) -> (-27.1153, -37.6879) projected
  line L622 (-27.1153, -37.6879) -> (-26.7611, -37.4792) projected
  line L623 (-26.7611, -37.4792) -> (-26.4145, -37.2644) projected
  line L624 (-26.4145, -37.2644) -> (-26.0759, -37.0434) projected
  line L625 (-26.0759, -37.0434) -> (-25.7456, -36.8158) projected
  line L626 (-25.7456, -36.8158) -> (-25.4241, -36.5817) projected
  line L627 (-25.4241, -36.5817) -> (-25.1121, -36.3405) projected
  line L628 (-25.1121, -36.3405) -> (-24.8101, -36.092) projected
  line L629 (-24.8101, -36.092) -> (-24.5194, -35.8356) projected
  line L630 (-24.5194, -35.8356) -> (-24.2415, -35.5701) projected
  line L631 (-24.2415, -35.5701) -> (-23.979, -35.294) projected
  line L632 (-23.979, -35.294) -> (-23.7394, -35.0022) projected
  line L633 (-23.7394, -35.0022) -> (-23.5736, -34.7774) projected
  line L634 (-23.5736, -34.7774) -> (-23.403, -34.5662) projected
  line L635 (-23.403, -34.5662) -> (-23.2294, -34.3678) projected
  line L636 (-23.2294, -34.3678) -> (-23.0555, -34.1805) projected
  line L637 (-23.0555, -34.1805) -> (-22.8765, -34.0078) projected
  line L638 (-22.8765, -34.0078) -> (-22.6925, -33.8498) projected
  line L639 (-22.6925, -33.8498) -> (-22.5034, -33.7069) projected
  line L640 (-22.5034, -33.7069) -> (-22.3146, -33.5758) projected
  line L641 (-22.3146, -33.5758) -> (-22.121, -33.4602) projected
  line L642 (-22.121, -33.4602) -> (-21.9209, -33.3615) projected
  line L643 (-21.9209, -33.3615) -> (-21.7207, -33.2758) projected
  line L644 (-21.7207, -33.2758) -> (-21.515, -33.2073) projected
  line L645 (-21.515, -33.2073) -> (-21.3046, -33.1558) projected
  line L646 (-21.3046, -33.1558) -> (-21.0926, -33.12) projected
  line L647 (-21.0926, -33.12) -> (-20.8729, -33.1046) projected
  line L648 (-20.8729, -33.1046) -> (-20.6524, -33.1063) projected
  line L649 (-20.6524, -33.1063) -> (-20.4215, -33.1323) projected
  line L650 (-20.4215, -33.1323) -> (-20.186, -33.1812) projected
  line L651 (-20.186, -33.1812) -> (-19.9271, -33.2679) projected
  line L652 (-19.9271, -33.2679) -> (-19.6145, -33.4191) projected
  line L653 (-19.6145, -33.4191) -> (-19.5667, -33.4471) projected
  line L654 (-19.5667, -33.4471) -> (-19.5188, -33.475) projected
  line L655 (-19.5188, -33.475) -> (-19.4709, -33.5029) projected
  line L656 (-19.4709, -33.5029) -> (-19.423, -33.5307) projected
  line L657 (-19.423, -33.5307) -> (-19.375, -33.5585) projected
  line L658 (-19.375, -33.5585) -> (-19.327, -33.5862) projected
  line L659 (-19.327, -33.5862) -> (-19.2789, -33.6138) projected
  line L660 (-19.2789, -33.6138) -> (-19.2308, -33.6413) projected
  line L661 (-19.2308, -33.6413) -> (-19.1827, -33.6688) projected
  line L662 (-19.1827, -33.6688) -> (-19.1345, -33.6962) projected
  line L663 (-19.1345, -33.6962) -> (-18.8473, -33.8913) projected
  line L664 (-18.8473, -33.8913) -> (-18.6427, -34.0722) projected
  line L665 (-18.6427, -34.0722) -> (-18.4826, -34.2517) projected
  line L666 (-18.4826, -34.2517) -> (-18.3447, -34.4386) projected
  line L667 (-18.3447, -34.4386) -> (-18.2329, -34.6288) projected
  line L668 (-18.2329, -34.6288) -> (-18.1365, -34.8267) projected
  line L669 (-18.1365, -34.8267) -> (-18.0614, -35.0282) projected
  line L670 (-18.0614, -35.0282) -> (-18.0008, -35.2362) projected
  line L671 (-18.0008, -35.2362) -> (-17.9574, -35.4486) projected
  line L672 (-17.9574, -35.4486) -> (-17.9314, -35.6648) projected
  line L673 (-17.9314, -35.6648) -> (-17.9169, -35.8874) projected
  line L674 (-17.9169, -35.8874) -> (-17.9202, -36.1129) projected
  line L675 (-17.9202, -36.1129) -> (-17.9393, -36.342) projected
  line L676 (-17.9393, -36.342) -> (-17.9685, -36.5772) projected
  line L677 (-17.9685, -36.5772) -> (-18.0133, -36.8155) projected
  line L678 (-18.0133, -36.8155) -> (-18.0734, -37.0569) projected
  line L679 (-18.0734, -37.0569) -> (-18.1486, -37.3012) projected
  line L680 (-18.1486, -37.3012) -> (-18.2337, -37.5507) projected
  line L681 (-18.2337, -37.5507) -> (-18.3313, -37.804) projected
  line L682 (-18.3313, -37.804) -> (-18.4431, -38.0601) projected
  line L683 (-18.4431, -38.0601) -> (-18.576, -38.4134) projected
  line L684 (-18.576, -38.4134) -> (-18.6839, -38.7788) projected
  line L685 (-18.6839, -38.7788) -> (-18.7748, -39.1522) projected
  line L686 (-18.7748, -39.1522) -> (-18.8516, -39.5322) projected
  line L687 (-18.8516, -39.5322) -> (-18.9158, -39.9179) projected
  line L688 (-18.9158, -39.9179) -> (-18.9686, -40.3088) projected
  line L689 (-18.9686, -40.3088) -> (-19.0107, -40.7043) projected
  line L690 (-19.0107, -40.7043) -> (-19.0425, -41.1041) projected
  line L691 (-19.0425, -41.1041) -> (-19.0647, -41.5079) projected
  line L692 (-19.0647, -41.5079) -> (-19.0774, -41.9154) projected
  line L693 (-19.0774, -41.9154) -> (-19.081, -42.3265) projected
  line L694 (-19.081, -42.3265) -> (-19.0757, -42.7409) projected
  line L695 (-19.0757, -42.7409) -> (-19.0617, -43.1585) projected
  line L696 (-19.0617, -43.1585) -> (-19.0392, -43.579) projected
  line L697 (-19.0392, -43.579) -> (-19.0083, -44.0023) projected
  line L698 (-19.0083, -44.0023) -> (-18.969, -44.4283) projected
  line L699 (-18.969, -44.4283) -> (-18.9216, -44.8569) projected
  line L700 (-18.9216, -44.8569) -> (-18.866, -45.2878) projected
  line L701 (-18.866, -45.2878) -> (-18.8024, -45.721) projected
  line L702 (-18.8024, -45.721) -> (-18.7309, -46.1563) projected
  line L703 (-18.7309, -46.1563) -> (-18.394, -46.2916) projected
  line L704 (-18.394, -46.2916) -> (-18.0561, -46.4245) projected
  line L705 (-18.0561, -46.4245) -> (-17.7172, -46.5548) projected
  line L706 (-17.7172, -46.5548) -> (-17.3775, -46.6827) projected
  line L707 (-17.3775, -46.6827) -> (-17.0368, -46.8081) projected
  line L708 (-17.0368, -46.8081) -> (-16.6952, -46.9311) projected
  line L709 (-16.6952, -46.9311) -> (-16.3527, -47.0515) projected
  line L710 (-16.3527, -47.0515) -> (-16.0093, -47.1694) projected
  line L711 (-16.0093, -47.1694) -> (-15.6651, -47.2849) projected
  line L712 (-15.6651, -47.2849) -> (-15.32, -47.3978) projected
  line L713 (-15.32, -47.3978) -> (-14.9854, -47.1103) projected
  line L714 (-14.9854, -47.1103) -> (-14.6582, -46.8193) projected
  line L715 (-14.6582, -46.8193) -> (-14.3387, -46.5249) projected
  line L716 (-14.3387, -46.5249) -> (-14.0269, -46.2271) projected
  line L717 (-14.0269, -46.2271) -> (-13.723, -45.926) projected
  line L718 (-13.723, -45.926) -> (-13.4272, -45.6216) projected
  line L719 (-13.4272, -45.6216) -> (-13.1396, -45.314) projected
  line L720 (-13.1396, -45.314) -> (-12.8605, -45.0031) projected
  line L721 (-12.8605, -45.0031) -> (-12.59, -44.689) projected
  line L722 (-12.59, -44.689) -> (-12.3286, -44.3718) projected
  line L723 (-12.3286, -44.3718) -> (-12.0764, -44.0514) projected
  line L724 (-12.0764, -44.0514) -> (-11.8338, -43.7278) projected
  line L725 (-11.8338, -43.7278) -> (-11.6012, -43.4011) projected
  line L726 (-11.6012, -43.4011) -> (-11.3792, -43.0711) projected
  line L727 (-11.3792, -43.0711) -> (-11.1684, -42.7378) projected
  line L728 (-11.1684, -42.7378) -> (-10.9697, -42.401) projected
  line L729 (-10.9697, -42.401) -> (-10.7842, -42.0605) projected
  line L730 (-10.7842, -42.0605) -> (-10.6138, -41.716) projected
  line L731 (-10.6138, -41.716) -> (-10.4616, -41.3668) projected
  line L732 (-10.4616, -41.3668) -> (-10.3363, -41.0107) projected
  line L733 (-10.3363, -41.0107) -> (-10.2968, -40.8767) projected
  line L734 (-10.2968, -40.8767) -> (-9.3826, -37.2474) projected
  arc A5 (-9.0329, -36.5223) -> (-9.3826, -37.2474) centre (-7.4432, -37.7359) ccw projected
  line L735 (-9.0329, -36.5223) -> (11.4682, -9.6686) projected
  line L736 (11.4682, -9.6686) -> (33.8389, 16.8659) projected
  arc A6 (34.1366, 17.1528) -> (33.8389, 16.8659) centre (35.368, 15.5768) ccw projected
  line L737 (34.1366, 17.1528) -> (50.1161, 29.6374) projected
  arc A7 (50.1161, 29.6374) -> (50.5705, 32.2897) centre (48.8848, 31.2134) ccw projected
  arc A8 (50.5705, 32.2897) -> (43.5647, 41.2567) centre (0, 0) ccw projected
  arc A9 (43.5647, 41.2567) -> (40.8812, 41.4575) centre (42.1125, 39.8815) ccw projected
  line L738 (40.8812, 41.4575) -> (18.4224, 23.9108) projected
  arc A10 (15.2685, 26.0381) -> (18.4224, 23.9108) centre (17.1911, 25.4868) ccw projected
  line L739 (15.2685, 26.0381) -> (23.1244, 53.4347) projected
  arc A11 (-27.4643, 16.414) -> (-12.9468, -29.2349) centre (0.018, 0.0211) ccw projected
  arc A12 (-24.4501, 16.9123) -> (-27.4643, 16.414) centre (-25.7466, 15.3894) ccw projected
  line L740 (-24.4501, 16.9123) -> (-14.2985, 8.2696) projected
  arc A13 (-13.7582, 5.9555) -> (-14.2985, 8.2696) centre (-15.595, 6.7468) ccw projected
  arc A14 (-13.7582, 5.9555) -> (-3.384, -14.588) centre (0.018, 0.0211) ccw projected
  arc A15 (-2.2479, -17.7495) -> (-3.384, -14.588) centre (-3.8376, -16.5359) ccw projected
  line L741 (-2.2479, -17.7495) -> (-10.5468, -28.62) projected
  arc A16 (-12.9468, -29.2349) -> (-10.5468, -28.62) centre (-12.1365, -27.4064) ccw projected
  arc A17 (-4.6156, 14.2875) -> (-8.0384, 12.674) centre (0.018, 0.0211) ccw projected
  arc A18 (-10.409, 12.8382) -> (-8.0384, 12.674) centre (-9.1125, 14.3611) ccw projected
  line L742 (-10.409, 12.8382) -> (-20.5607, 21.4809) projected
  arc A19 (-20.5496, 24.5359) -> (-20.5607, 21.4809) centre (-19.2642, 23.0037) ccw projected
  arc A20 (-18.5954, 26.0508) -> (-20.5496, 24.5359) centre (0.018, 0.0211) ccw projected
  arc A21 (-18.209, 26.2668) -> (-18.5954, 26.0508) centre (-17.432, 24.4239) ccw projected
  line L743 (-18.209, 26.2668) -> (-1.6471, 33.2492) projected
  arc A22 (1.0524, 30.855) -> (-1.6471, 33.2492) centre (-0.8702, 31.4063) ccw projected
  line L744 (1.0524, 30.855) -> (-3.3109, 15.6384) projected
  arc A23 (-4.6156, 14.2875) -> (-3.3109, 15.6384) centre (-5.2335, 16.1897) ccw projected
  circle A24 centre (13.5062, 47.1018) radius 1.2295 projected
  circle A25 centre (38.6125, 30.1674) radius 1.2295 projected
  circle A26 centre (26.7924, 20.9325) radius 1.2295 projected
  circle A27 centre (9.3717, 32.6829) radius 1.2295 projected
  circle A28 centre (0, 0) radius 9.5 projected
  arc A29 (11.4682, -9.6686) -> (11.4864, 9.6469) centre (0, 0) ccw
  circle A30 centre (0, 0) radius 9.5 projected
  arc A31 (-13.7582, 5.9555) -> (-3.384, -14.588) centre (0.018, 0.0211) ccw projected
  line L745 (15.2685, 26.0381) -> (11.0954, 11.4845)
  line L746 (15.2685, 26.0381) -> (23.1244, 53.4347) projected
  arc A32 (11.0954, 11.4845) -> (11.4864, 9.6469) centre (13.0179, 10.9332) ccw
  point P0 (10.7901, 10.4199)
  dimension "d46" = 2
  constraints: 5 point on circle, 2 centre point, 2 end point, 2 point on line, 2 tangent, 1 collinear, 1 concentric, 1 equal radius
  measures "d46" radius of A32
extrude "押し出し6" cut sketch "スケッチ6" against normal through all contours A10 L738 A9 A8 A7 L737 A6 L736 A29 A32 L745
